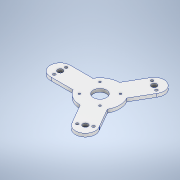
# Autodesk Inventor part: De_Duoi
Saved by Autodesk Inventor 2022 (Build 260153000, 153)
## iProperties
Created: 2022-11-10
Part Number: De_Duoi
Material: Aluminum 6061
Document SubType Name: Modeling
Designer: nguye
Density: 2.7 g/cm^3
Appearance: Aluminum - Flat
Author: nguye
Autodesk Inventor part; units mm, degrees
ref_plane "YZ Plane" through (0, 0, 0) normal (1, 0, 0) x (0, 1, 0)
ref_plane "XZ Plane" through (0, 0, 0) normal (0, 1, 0) x (-1, 0, 0)
ref_plane "XY Plane" through (0, 0, 0) normal (0, 0, 1) x (1, 0, 0)
sketch "Sketch1" plane through (0, 0, 0) normal (0, 1, 0) x (-1, 0, 0)
  circle A0 centre (0, 0) radius 60
  circle A1 centre (60, 0) radius 4
  circle A2 centre (-30, 51.9615) radius 4
  circle A3 centre (-30, -51.9615) radius 4
  circle A4 centre (-30, 51.9615) radius 15
  circle A5 centre (-30, -51.9615) radius 15
  circle A6 centre (60, 0) radius 15
  line L0 (21, -21) -> (-21, -21)
  line L1 (-21, -21) -> (-21, 21)
  line L2 (-21, 21) -> (21, 21)
  line L3 (21, 21) -> (21, -21)
  line L4 (21, -21) -> (-21, 21) construction
  line L5 (-21, -21) -> (21, 21) construction
  line L6 (67.5, 12.9904) -> (-22.5, 64.9519)
  line L7 (67.5, -12.9904) -> (-22.5, -64.9519)
  line L8 (-45, 51.9615) -> (-45, -51.9615)
  circle A7 centre (0, 0) radius 10
  line L9 (67.5, 12.9904) -> (21, 39.8372)
  line L10 (60, 15) -> (25.632, 15)
  line L11 (60, -15) -> (25.632, -15)
  circle A8 centre (0, 0) radius 29.6985
  circle A9 centre (28.3546, 20) radius 5
  circle A10 centre (28.3546, -20) radius 5
  circle A11 centre (-31.4978, 14.5558) radius 5
  line L12 (-42.9904, 44.4615) -> (-25.8064, 14.698)
  line L13 (-17.0096, 59.4615) -> (0.1744, 29.698)
  circle A12 centre (3.1432, 34.5558) radius 5
  circle A13 centre (3.1432, -34.5558) radius 5
  line L14 (-17.0096, -59.4615) -> (0.1744, -29.698)
  line L15 (-42.9904, -44.4615) -> (-25.8064, -14.698)
  circle A14 centre (-31.4978, -14.5558) radius 5
  point P0 (16, -16)
  point P1 (16, 16)
  point P2 (-16, 16)
  point P3 (-16, -16)
  point P4 (-16.174, 57.7789)
  point P5 (-41.951, 42.8966)
  point P6 (-42.0378, 42.8115)
  point P7 (-25.8064, 14.698)
  point P8 (-25.8064, -14.698)
  point P9 (-42.0378, -42.8115)
  point P10 (-41.951, -42.8966)
  point P11 (-16.174, -57.7789)
  point P12 (-16.057, -57.8115)
  point P13 (58.0948, -15)
  point P14 (58.125, -14.8824)
  point P15 (58.125, 14.8824)
  point P16 (58.0948, 15)
  point P17 (-16.057, 57.8115)
  dimension "d0" = 120
  dimension "d2" = 8
  dimension "d5" = 360
  dimension "d7" = 30
  dimension "d8" = 30
  dimension "d9" = 30
  dimension "d10" = 42
  dimension "d11" = 42
  dimension "d12" = 20
  dimension "d13" = 32
  dimension "d14" = 16
  dimension "d15" = 16
  dimension "d16" = 32
  dimension "d17" = 10
  dimension "d18" = 10
  dimension "d21" = 360
  constraints: 32 end point, 14 centre point, 12 tangent, 11 point on circle, 6 coincident, 3 horizontal alignment, 3 perpendicular, 3 vertical alignment, 2 midpoint, 2 parallel, 1 horizontal, 1 point on line, 41 other
  measures "d2" diameter of A1
  measures "d7" diameter of A4
  measures "d8" diameter of A5
  measures "d9" diameter of A6
  measures "d10" distance of L1.end L2.end
  measures "d11" distance of L0.end L1.end
  measures "d12" diameter of A7
  measures "d13" distance of point (16, -16) point (16, 16)
  measures "d14" horizontal distance of point (16, -16) point (0, 0)
  measures "d15" horizontal distance of point (16, -16) point (0, 0)
  measures "d16" distance of point (16, 16) point (-16, 16)
  measures "d17" diameter of A9
  measures "d18" diameter of A10
extrude "Extrusion1" add sketch "Sketch1" along normal blind 5 contours A1 A0 A6 | A0 A6 A1 | A6 A0 L11 A8 L10 | A8 L3 | L13 A8 L12 A0 A4 | A4 A0 A2 | L3 L0 L1 L2 | L2 A8 | A0 A5 L15 A8 L14 | A5 A0 A3 | A8 L0 | A4 A0 A2 | L1 A8 | A0 A3 A5
sketch "Sketch2" plane through (0, 5, 0) normal (0, 1, 0) x (1, 0, 0)
  point P0 (0, 0)
  point P1 (-15.5, -15.5)
  point P2 (-15.5, 15.5)
  point P3 (15.5, -15.5)
  point P4 (15.5, 15.5)
  dimension "d25" = 31
  dimension "d26" = 31
  dimension "d27" = 15.5
  dimension "d28" = 15.5
  constraints: 2 horizontal alignment, 2 vertical alignment
  measures "d25" distance of point (-15.5, 15.5) point (-15.5, -15.5)
  measures "d26" distance of point (-15.5, 15.5) point (15.5, 15.5)
  measures "d27" horizontal distance of point (-15.5, 15.5) point (0, 0)
  measures "d28" horizontal distance of point (-15.5, 15.5) point (0, 0)
hole "Hole1" at (-15.5, 5, 15.5) at (-15.5, 5, -15.5) at (15.5, 5, 15.5) at (15.5, 5, -15.5) direction (0, -1, 0) diameter 3.05 end through all
sketch "Sketch3" plane through (0, 5, 0) normal (0, 1, 0) x (1, 0, 0)
  circle A0 centre (-60, 0) radius 4 projected
  point P0 (0, 0)
  point P1 (-60, -9)
  point P2 (-60, 9)
  dimension "d36" = 9
  dimension "d37" = 18
  constraints: 2 vertical alignment
  measures "d36" distance of A0.centre point (-60, -9)
  measures "d37" distance of point (-60, 9) point (-60, -9)
hole "Hole2" at (-60, 5, 9) at (-60, 5, -9) direction (0, -1, 0) diameter 4 end through all
pattern_circular "Circular Pattern1" count 3 over 360 about axis through (0, 0, 0) along (0, 1, 0) of "Hole2"
body "Solid1"
